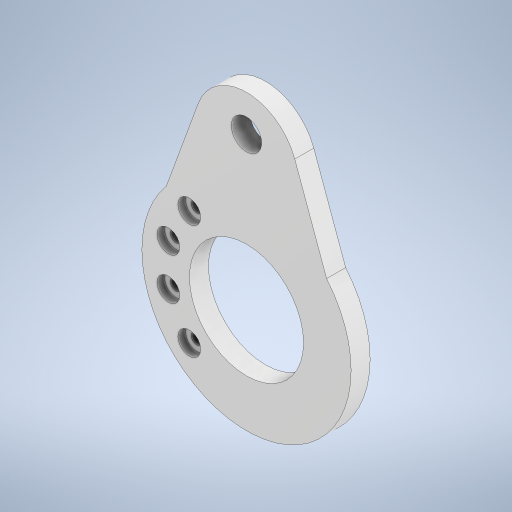
# Autodesk Inventor part: legparts_04(seven)
Saved by Autodesk Inventor 2024.3 (Build 283343000, 343)
## iProperties
Created: 2024-10-20
Part Number: legparts_04(seven)
Material: ABS プラスチック
Document SubType Name: Modeling
Designer: 佐藤智貴
Density: 1.06 g/cm^3
Appearance: 滑らか - 白
Mass: 11.7138 g
Surface Area: 63.8288 cm^2
Volume: 11.0508 cm^3
Author: 佐藤智貴
Autodesk Inventor part; units mm, degrees
ref_plane "YZ Plane" through (0, 0, 0) normal (1, 0, 0) x (0, 1, 0)
ref_plane "XZ Plane" through (0, 0, 0) normal (0, 1, 0) x (-1, 0, 0)
ref_plane "XY Plane" through (0, 0, 0) normal (0, 0, 1) x (1, 0, 0)
sketch "スケッチ12" plane through (0, 0, 0) normal (0, 0, 1) x (1, 0, 0)
  circle A0 centre (0, 0) radius 27.5
  circle A1 centre (0, 0) radius 15
  line L0 (-27.5, 0) -> (27.5, 0)
  line L1 (-27.5, 0) -> (-9.3015, 50)
  line L2 (-9.3015, 50) -> (9.3015, 50)
  line L3 (9.3015, 50) -> (27.5, 0)
  circle A2 centre (0, 40) radius 4
  line L4 (9.3015, 50) -> (-27.5, 0)
  line L5 (-9.3015, 50) -> (27.5, 0)
  point P0 (21.0662, 17.6767)
  point P1 (-21.0662, 17.6767)
  point P2 (0, 51.9615)
  point P3 (8.174, 26.2571)
  point P4 (-8.174, 26.2571)
  point P5 (-2.2669, 48.0351)
  point P6 (2.2669, 48.0351)
  point P7 (0, 37.3626)
  point P8 (-15, 0)
  point P9 (15, 0)
  dimension "d5" = 55
  dimension "d6" = 30
  dimension "d10" = 70
  dimension "d11" = 70
  dimension "d12" = 50
  dimension "d13" = 40
  dimension "d14" = 8
  dimension "d47" = 0
  constraints: 12 end point, 3 centre point, 2 horizontal, 2 point on circle, 1 coincident, 1 midpoint
  measures "d5" diameter of A0
  measures "d6" diameter of A1
  measures "d10" angle of L0 L3
  measures "d11" angle of L0 L1
  measures "d12" distance between parallel lines of L0 L2
  measures "d13" distance from line of L0 A2.centre
  measures "d14" diameter of A2
  measures "d47" horizontal distance of point (0, 0) A2.centre
extrude "押し出し2" add sketch "スケッチ12" along normal blind 5 contours L0 A1 A0 | L4 A0 L5 L0 A1 | A0 L1 | L1 A0 L4 | L3 A0 | L5 A0 L3 | L1 L5 A2 L4 A0 | L4 A2 L5 A0 | A0 L5 A2 L4 L3 | L2 L4 A2 L5
sketch "スケッチ13" plane through (0, 0, 5) normal (0, 0, 1) x (1, 0, 0)
  circle A0 centre (0, 0) radius 17.5
  circle A1 centre (0, 0) radius 25
  circle A2 centre (0, 0) radius 21.25
  line L0 (0, 0) -> (-18.638, 32.282)
  line L1 (-18.638, 32.282) -> (0, 0)
  line L2 (0, 0) -> (-17.2844, -29.9374)
  line L3 (0, 0) -> (-56.8729, 0)
  line L4 (0, 0) -> (-31.7394, -18.3248)
  line L5 (0, 0) -> (-33.3883, 19.2767)
  line L6 (0, 0) -> (0, -31.9785)
  line L7 (0, 0) -> (-25.7143, 25.7143)
  line L8 (0, 0) -> (-33.0547, 8.857)
  line L9 (0, 0) -> (-32.621, -8.7408)
  line L10 (0, 0) -> (-23.652, -23.652)
  point P0 (-18.403, 10.625)
  point P1 (-21.25, 0)
  point P2 (-18.403, -10.625)
  point P3 (-10.625, -18.403)
  point P4 (0, -21.25)
  point P5 (-16.5273, 4.4285)
  point P6 (-15.026, 15.026)
  point P7 (-20.5259, 5.4999)
  point P8 (-20.5259, -5.4999)
  point P9 (-15.026, -15.026)
  dimension "d19" = 42.5
  dimension "d17" = 35
  dimension "d18" = 50
  dimension "d20" = 60
  dimension "d21" = 60
  dimension "d22" = 30
  dimension "d23" = 30
  dimension "d31" = 150
  dimension "d32" = 15
  dimension "d34" = 15
  dimension "d35" = 15
  dimension "d36" = 15
  constraints: 22 end point, 9 point on line, 2 centre point, 1 coincident, 1 collinear, 1 horizontal, 1 midpoint, 1 vertical, 11 other
  measures "d17" diameter of A0
  measures "d18" diameter of A1
  measures "d20" angle of L3 L0
  measures "d21" angle of L2 L3
  measures "d22" angle of L2 L4
  measures "d23" angle of L3 L5
  measures "d31" angle of L6 L0
  measures "d32" angle of L0 L7
  measures "d34" angle of L8 L5
  measures "d35" angle of L3 L9
  measures "d36" angle of L4 L10
hole "穴1" at (-15.026, 15.026, 5) at (-20.5259, 5.4999, 5) at (-20.5259, -5.4999, 5) at (-15.026, -15.026, 5) direction (0, 0, -1) diameter 3 end through all
sketch "スケッチ14" plane through (0, 0, 5) normal (0, 0, 1) x (1, 0, 0)
  circle A0 centre (-15.026, 15.026) radius 1.5 projected
  circle A1 centre (-15.026, 15.026) radius 3
  circle A2 centre (-20.5259, 5.4999) radius 1.5 projected
  circle A3 centre (-20.5259, 5.4999) radius 3
  circle A4 centre (-20.5259, -5.4999) radius 1.5 projected
  circle A5 centre (-20.5259, -5.4999) radius 3
  circle A6 centre (-15.026, -15.026) radius 1.5 projected
  circle A7 centre (-15.026, -15.026) radius 3
  point P0 (0, 0)
  dimension "d40" = 6
  dimension "d41" = 6
  dimension "d42" = 6
  dimension "d43" = 6
  constraints: 4 centre point, 4 coincident
  measures "d40" diameter of A1
  measures "d41" diameter of A3
  measures "d42" diameter of A5
  measures "d43" diameter of A7
extrude "押し出し3" cut sketch "スケッチ14" against normal blind 2 contours A0 | A1 | A2 | A3 | A4 | A5 | A6 | A7
fillet "フィレット3" radius 13.5 2 edges at (9.3015, 50, 2.5) (-9.3015, 50, 2.5)
equation "\"d10\" = d11"
equation "\"d35\" = d34"
equation "\"d36\" = d35"
equation "\"d41\" = d40"
equation "\"d42\" = d41"
equation "\"d43\" = d42"
